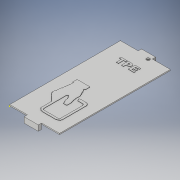
# Autodesk Inventor part: Pièce2
Saved by Autodesk Inventor 2017 (Build 210142000, 142)
## iProperties
Created: 2020-03-28
Part Number: Pièce2
Material: Generic
Document SubType Name: Modeling
Designer: LUC
Density: 1 g/cm^3
Appearance: Default
Author: LUC
Autodesk Inventor part; units mm, degrees
ref_plane "YZ Plane" through (0, 0, 0) normal (1, 0, 0) x (0, 1, 0)
ref_plane "XZ Plane" through (0, 0, 0) normal (0, 1, 0) x (-1, 0, 0)
ref_plane "XY Plane" through (0, 0, 0) normal (0, 0, 1) x (1, 0, 0)
sketch "Esquisse1" plane through (0, 0, 0) normal (0, 1, 0) x (-1, 0, 0)
  point P0 (0, 0)
sketch "Esquisse2" plane through (0, 0, 0) normal (0, 1, 0) x (-1, 0, 0)
  line L0 (0, 0) -> (-45, 0)
  line L1 (-45, 0) -> (-45, -100)
  line L2 (-45, -100) -> (0, -100)
  line L3 (0, -100) -> (0, 0)
  line L4 (-17.07, 0) -> (-29.07, 0)
  line L5 (-17.03, -100) -> (-29.03, -100)
  dimension "d0" = 45
  dimension "d1" = 100
  constraints: 12 end point, 3 horizontal, 2 parallel, 2 point on line, 1 perpendicular
  measures "d0" distance of L2.end L1.end
  measures "d1" distance of L1.end L0.end
extrude "Extrusion1" add sketch "Esquisse2" along normal blind 1
sketch "Esquisse5" plane through (0, 1, 0) normal (0, 1, 0) x (1, 0, 0)
  line L0 (4.5597, 87.1322) -> (40.1621, 87.1322) construction
  line L1 (40.1621, 87.1322) -> (40.1621, 77.2581) construction
  line L2 (40.1621, 77.2581) -> (4.5597, 77.2581) construction
  line L3 (4.5597, 77.2581) -> (4.5597, 87.1322) construction
  line L4 (13.3166, 87.1322) -> (19.0526, 87.1322)
  line L5 (19.0526, 87.1322) -> (19.0526, 85.6234)
  line L6 (19.0526, 85.6234) -> (17.1269, 85.6234)
  line L7 (17.1269, 85.6234) -> (17.1269, 81.0322)
  line L8 (17.1269, 81.0322) -> (15.2423, 81.0322)
  line L9 (15.2423, 81.0322) -> (15.2423, 85.6234)
  line L10 (15.2423, 85.6234) -> (13.3166, 85.6234)
  line L11 (13.3166, 85.6234) -> (13.3166, 87.1322)
  line L12 (19.898, 87.1322) -> (23.0332, 87.1322)
  spline S0 degree 2 poles (23.0332, 87.1322) (24.0547, 87.1322) (25.0763, 86.1576) (25.0763, 85.2594) knots 0 0 0 1 2 2 2
  spline S1 degree 2 poles (25.0763, 85.2594) (25.0763, 84.3317) (23.9667, 83.2926) (22.8277, 83.2926) knots 0 0 0 1 2 2 2
  line L13 (22.8277, 83.2926) -> (21.7944, 83.2926)
  line L14 (21.7944, 83.2926) -> (21.7944, 81.0322)
  line L15 (21.7944, 81.0322) -> (19.898, 81.0322)
  line L16 (19.898, 81.0322) -> (19.898, 87.1322)
  line L17 (21.7944, 84.5313) -> (22.2523, 84.5313)
  spline S2 degree 2 poles (22.2523, 84.5313) (22.7983, 84.5313) (23.2386, 84.913) (23.2386, 85.2065) knots 0 0 0 1 2 2 2
  spline S3 degree 2 poles (23.2386, 85.2065) (23.2386, 85.4942) (22.857, 85.8934) (22.3286, 85.8934) knots 0 0 0 1 2 2 2
  line L18 (22.3286, 85.8934) -> (21.7944, 85.8934)
  line L19 (21.7944, 85.8934) -> (21.7944, 84.5313)
  line L20 (26.0626, 87.1322) -> (31.1117, 87.1322)
  line L21 (31.1117, 87.1322) -> (31.1117, 85.8288)
  line L22 (31.1117, 85.8288) -> (27.9531, 85.8288)
  line L23 (27.9531, 85.8288) -> (27.9531, 84.8601)
  line L24 (27.9531, 84.8601) -> (30.8827, 84.8601)
  line L25 (30.8827, 84.8601) -> (30.8827, 83.6155)
  line L26 (30.8827, 83.6155) -> (27.9531, 83.6155)
  line L27 (27.9531, 83.6155) -> (27.9531, 82.4119)
  line L28 (27.9531, 82.4119) -> (31.2056, 82.4119)
  line L29 (31.2056, 82.4119) -> (31.2056, 81.0322)
  line L30 (31.2056, 81.0322) -> (26.0626, 81.0322)
  line L31 (26.0626, 81.0322) -> (26.0626, 87.1322)
  point P0 (0, 0)
  constraints: 2 other
sketch "Esquisse7" plane through (0, 1, 0) normal (0, 1, 0) x (1, 0, 0)
  line L0 (21.7399, 49.8058) -> (11.605, 49.8058)
  line L1 (11.605, 49.8058) -> (11.605, 49.5446)
  line L2 (11.605, 49.5446) -> (11.309, 49.5446)
  line L3 (11.309, 49.5446) -> (11.309, 49.1789)
  line L4 (11.309, 49.1789) -> (10.9955, 49.1789)
  line L5 (10.9955, 49.1789) -> (10.9955, 45.9399)
  line L6 (10.9955, 45.9399) -> (11.309, 45.9399)
  line L7 (11.309, 45.9399) -> (11.309, 45.6439)
  line L8 (11.309, 45.6439) -> (11.9185, 45.6439)
  line L9 (11.9185, 45.6439) -> (11.9185, 42.4572)
  line L10 (11.9185, 42.4572) -> (11.605, 42.4572)
  line L11 (11.605, 42.4572) -> (11.605, 40.5939)
  line L12 (11.605, 40.5939) -> (11.309, 40.5939)
  line L13 (11.309, 40.5939) -> (11.309, 38.6435)
  line L14 (11.309, 38.6435) -> (10.9955, 38.6435)
  line L15 (10.9955, 38.6435) -> (10.9955, 36.7595)
  line L16 (10.9955, 36.7595) -> (10.9955, 36.3411)
  line L17 (10.9955, 36.3411) -> (10.6437, 36.3411)
  line L18 (10.6437, 36.3411) -> (10.6437, 34.6078)
  line L19 (10.6437, 34.6078) -> (10.315, 34.6078)
  line L20 (10.315, 34.6078) -> (10.315, 32.9043)
  line L21 (10.315, 32.9043) -> (10.315, 31.5295)
  line L22 (10.315, 31.5295) -> (10.046, 31.5295)
  line L23 (10.046, 31.5295) -> (10.046, 30.9617)
  line L24 (10.046, 30.9617) -> (9.6276, 30.9617)
  line L25 (9.6276, 30.9617) -> (9.6276, 28.5111)
  line L26 (9.6276, 28.5111) -> (10.046, 28.5111)
  line L27 (10.046, 28.5111) -> (10.046, 28.003)
  line L28 (10.046, 28.003) -> (10.315, 28.003)
  line L29 (10.315, 28.003) -> (10.315, 27.3754)
  line L30 (10.315, 27.3754) -> (10.6437, 27.3754)
  line L31 (10.6437, 27.3754) -> (10.6437, 26.957)
  line L32 (10.6437, 26.957) -> (10.9955, 26.957)
  line L33 (10.9955, 26.957) -> (10.9955, 26.5984)
  line L34 (10.9955, 26.5984) -> (11.309, 26.5984)
  line L35 (11.309, 26.5984) -> (11.309, 26.1755)
  line L36 (11.309, 26.1755) -> (11.605, 26.1755)
  line L37 (11.605, 26.1755) -> (11.605, 25.8759)
  line L38 (11.605, 25.8759) -> (11.9185, 25.8759)
  line L39 (11.9185, 25.8759) -> (11.9185, 25.5291)
  line L40 (11.9185, 25.5291) -> (12.2466, 25.5291)
  line L41 (12.2466, 25.5291) -> (12.2466, 25.2575)
  line L42 (12.2466, 25.2575) -> (12.5562, 25.2575)
  line L43 (12.5562, 25.2575) -> (12.5562, 24.9339)
  line L44 (12.5562, 24.9339) -> (12.9079, 24.9339)
  line L45 (12.9079, 24.9339) -> (12.9079, 24.6525)
  line L46 (12.9079, 24.6525) -> (13.2175, 24.6525)
  line L47 (13.2175, 24.6525) -> (13.2175, 24.3007)
  line L48 (13.2175, 24.3007) -> (13.5411, 24.3007)
  line L49 (13.5411, 24.3007) -> (13.5411, 24.0193)
  line L50 (13.5411, 24.0193) -> (13.8225, 24.0193)
  line L51 (13.8225, 24.0193) -> (13.8225, 23.6957)
  line L52 (13.8225, 23.6957) -> (14.1883, 23.6957)
  line L53 (14.1883, 23.6957) -> (14.1883, 23.3862)
  line L54 (14.1883, 23.3862) -> (14.4979, 23.3862)
  line L55 (14.4979, 23.3862) -> (14.4979, 23.1329)
  line L56 (14.4979, 23.1329) -> (14.8074, 23.1329)
  line L57 (14.8074, 23.1329) -> (14.8074, 22.7389)
  line L58 (14.8074, 22.7389) -> (15.1029, 22.7389)
  line L59 (15.1029, 22.7389) -> (15.1029, 22.3872)
  line L60 (15.1029, 22.3872) -> (15.4687, 22.3872)
  line L61 (15.4687, 22.3872) -> (15.4687, 22.1058)
  line L62 (15.4687, 22.1058) -> (15.7501, 22.1058)
  line L63 (15.7501, 22.1058) -> (15.7501, 21.7399)
  line L64 (15.7501, 21.7399) -> (16.0878, 21.7399)
  line L65 (16.0878, 21.7399) -> (16.0878, 21.4304)
  line L66 (16.0878, 21.4304) -> (16.327, 21.4304)
  line L67 (16.327, 21.4304) -> (16.327, 21.1349)
  line L68 (16.327, 21.1349) -> (16.6724, 21.1349)
  line L69 (16.6724, 21.1349) -> (16.6724, 11.3222)
  line L70 (16.6724, 11.3222) -> (16.9934, 11.3222)
  line L71 (16.9934, 11.3222) -> (16.9934, 10.929)
  line L72 (16.9934, 10.929) -> (17.3843, 10.929)
  line L73 (17.3843, 10.929) -> (17.3843, 10.5721)
  line L74 (17.3843, 10.5721) -> (17.6902, 10.5721)
  line L75 (17.6902, 10.5721) -> (17.6902, 10.2832)
  line L76 (17.6902, 10.2832) -> (18.0641, 10.2832)
  line L77 (18.0641, 10.2832) -> (18.0641, 9.9943)
  line L78 (18.0641, 9.9943) -> (18.387, 9.9943)
  line L79 (18.387, 9.9943) -> (18.387, 9.6714)
  line L80 (18.387, 9.6714) -> (18.625, 9.6714)
  line L81 (18.625, 9.6714) -> (18.625, 9.3825)
  line L82 (18.625, 9.3825) -> (19.9166, 9.3825)
  line L83 (19.9166, 9.3825) -> (19.9166, 9.0596)
  line L84 (19.9166, 9.0596) -> (32.793, 9.0596)
  line L85 (32.793, 9.0596) -> (32.793, 9.3825)
  line L86 (32.793, 9.3825) -> (33.9518, 9.3825)
  line L87 (33.9518, 9.3825) -> (33.9518, 9.6714)
  line L88 (33.9518, 9.6714) -> (34.4661, 9.6714)
  line L89 (34.4661, 9.6714) -> (34.4661, 9.9943)
  line L90 (34.4661, 9.9943) -> (34.8776, 9.9943)
  line L91 (34.8776, 9.9943) -> (34.8776, 10.2832)
  line L92 (34.8776, 10.2832) -> (35.2634, 10.2832)
  line L93 (35.2634, 10.2832) -> (35.2634, 10.5721)
  line L94 (35.2634, 10.5721) -> (35.5205, 10.5721)
  line L95 (35.5205, 10.5721) -> (35.5205, 10.7506)
  line L96 (35.5205, 10.7506) -> (35.5205, 11.5083)
  line L97 (35.5205, 11.5083) -> (35.8034, 11.5083)
  line L98 (35.8034, 11.5083) -> (35.8034, 33.8684)
  line L99 (35.8034, 33.8684) -> (35.5205, 33.8684)
  line L100 (35.5205, 33.8684) -> (35.5205, 34.6078)
  line L101 (35.5205, 34.6078) -> (35.2634, 34.6078)
  line L102 (35.2634, 34.6078) -> (35.2634, 34.8498)
  line L103 (35.2634, 34.8498) -> (34.8776, 34.8498)
  line L104 (34.8776, 34.8498) -> (34.8776, 35.2086)
  line L105 (34.8776, 35.2086) -> (34.6719, 35.2086)
  line L106 (34.6719, 35.2086) -> (34.6719, 35.4745)
  line L107 (34.6719, 35.4745) -> (33.3724, 35.4745)
  line L108 (33.3724, 35.4745) -> (33.3724, 35.8589)
  line L109 (33.3724, 35.8589) -> (27.4994, 35.8589)
  line L110 (27.4994, 35.8589) -> (27.4994, 35.4745)
  line L111 (27.4994, 35.4745) -> (27.1406, 35.4745)
  line L112 (27.1406, 35.4745) -> (27.1406, 35.0292)
  line L113 (27.1406, 35.0292) -> (27.4994, 35.0292)
  line L114 (27.4994, 35.0292) -> (27.4994, 33.8684)
  line L115 (28.06, 33.8684) -> (28.1721, 33.4596)
  line L116 (28.1721, 33.4596) -> (32.9708, 33.4596)
  line L117 (32.9708, 33.4596) -> (32.9708, 33.2578)
  line L118 (32.9708, 33.2578) -> (33.2174, 33.2578)
  line L119 (33.2174, 33.2578) -> (33.2174, 32.9043)
  line L120 (33.2174, 32.9043) -> (33.6435, 32.9043)
  line L121 (33.6435, 32.9043) -> (33.6435, 32.2169)
  line L122 (33.6435, 32.2169) -> (33.9518, 32.2169)
  line L123 (33.9518, 32.2169) -> (33.9518, 11.8713)
  line L124 (33.9518, 11.8713) -> (33.6435, 11.8713)
  line L125 (33.6435, 11.8713) -> (33.6435, 11.2079)
  line L126 (33.6435, 11.2079) -> (33.2764, 11.2079)
  line L127 (33.2764, 11.2079) -> (33.2764, 10.929)
  line L128 (33.2764, 10.929) -> (19.5666, 10.929)
  line L129 (19.5666, 10.929) -> (19.5666, 11.2079)
  line L130 (19.5666, 11.2079) -> (19.2708, 11.2079)
  line L131 (19.2708, 11.2079) -> (19.2708, 11.5396)
  line L132 (19.2708, 11.5396) -> (18.9755, 11.5396)
  line L133 (18.9755, 11.5396) -> (18.9755, 12.1696)
  line L134 (18.9755, 12.1696) -> (18.625, 12.1696)
  line L135 (18.625, 12.1696) -> (18.625, 32.5606)
  line L136 (18.625, 32.5606) -> (18.9755, 32.5606)
  line L137 (18.9755, 32.5606) -> (18.9755, 32.9043)
  line L138 (18.9755, 32.9043) -> (18.9755, 33.2578)
  line L139 (18.9755, 33.2578) -> (19.5666, 33.2399)
  line L140 (19.5666, 33.2399) -> (19.5666, 33.5677)
  line L141 (19.5666, 33.5677) -> (19.8877, 33.5677)
  line L142 (19.8877, 33.5677) -> (19.8877, 32.9043)
  line L143 (19.8877, 32.9043) -> (20.1961, 32.9043)
  line L144 (20.1961, 32.9043) -> (20.1961, 32.5606)
  line L145 (20.1961, 32.5606) -> (20.5094, 32.5606)
  line L146 (20.5094, 32.5606) -> (20.5094, 31.9807)
  line L147 (20.5094, 31.9807) -> (21.149, 31.9807)
  line L148 (21.149, 31.9807) -> (21.149, 31.3486)
  line L149 (21.149, 31.3486) -> (21.5008, 31.3486)
  line L150 (21.5008, 31.3486) -> (21.5008, 30.6609)
  line L151 (21.5008, 30.6609) -> (21.784, 30.6609)
  line L152 (21.784, 30.6609) -> (21.784, 28.4465)
  line L153 (21.784, 28.4465) -> (22.1511, 28.4465)
  line L154 (22.1511, 28.4465) -> (22.1511, 27.5143)
  line L155 (22.1511, 27.5143) -> (22.4573, 27.5143)
  line L156 (22.4573, 27.5143) -> (22.4573, 26.871)
  line L157 (22.4573, 26.871) -> (22.7348, 26.871)
  line L158 (22.7348, 26.871) -> (22.7348, 26.5304)
  line L159 (22.7348, 26.5304) -> (23.088, 26.5304)
  line L160 (23.088, 26.5304) -> (23.088, 25.8759)
  line L161 (23.088, 25.8759) -> (23.416, 25.8759)
  line L162 (23.416, 25.8759) -> (23.416, 25.2575)
  line L163 (23.416, 25.2575) -> (23.7313, 25.2575)
  line L164 (23.7313, 25.2575) -> (23.7313, 24.9339)
  line L165 (23.7313, 24.9339) -> (26.2794, 24.9339)
  line L166 (26.2794, 24.9339) -> (26.2794, 25.5667)
  line L167 (26.2794, 25.5667) -> (26.5845, 25.5667)
  line L168 (26.5845, 25.5667) -> (26.5845, 29.0911)
  line L169 (26.5845, 29.0911) -> (26.2794, 29.0911)
  line L170 (26.2794, 29.0911) -> (26.2794, 30.3514)
  line L171 (26.2794, 30.3514) -> (25.9641, 30.3514)
  line L172 (25.9641, 30.3514) -> (25.9641, 31.6647)
  line L173 (25.9641, 31.6647) -> (25.5856, 31.6647)
  line L174 (25.5856, 31.6647) -> (25.5856, 33.8684)
  line L175 (25.5856, 33.8684) -> (25.2829, 33.8684)
  line L176 (25.2829, 33.8684) -> (25.2829, 38.6435)
  line L177 (25.2829, 38.6435) -> (25.0054, 38.6435)
  line L178 (25.0054, 38.6435) -> (25.0054, 39.2708)
  line L179 (25.0054, 39.2708) -> (24.6774, 39.2708)
  line L180 (24.6774, 39.2708) -> (24.6774, 40.3012)
  line L181 (24.6774, 40.3012) -> (24.4084, 40.3012)
  line L182 (24.4084, 40.3012) -> (24.4084, 40.9021)
  line L183 (24.4084, 40.9021) -> (24.0221, 40.9021)
  line L184 (24.0221, 40.9021) -> (24.0221, 41.2311)
  line L185 (24.0221, 41.2311) -> (23.7313, 41.2311)
  line L186 (23.7313, 41.2311) -> (23.7313, 41.8463)
  line L187 (23.7313, 41.8463) -> (23.416, 41.8463)
  line L188 (23.416, 41.8463) -> (23.416, 42.8192)
  line L189 (23.416, 42.8192) -> (23.088, 42.8192)
  line L190 (23.088, 42.8192) -> (23.088, 43.1196)
  line L191 (23.088, 43.1196) -> (22.7348, 43.1196)
  line L192 (22.7348, 43.1196) -> (22.7348, 43.7491)
  line L193 (22.7348, 43.7491) -> (22.4573, 43.7491)
  line L194 (22.4573, 43.7491) -> (22.4573, 44.0505)
  line L195 (22.4573, 44.0505) -> (22.1511, 44.0505)
  line L196 (22.1511, 44.0505) -> (22.1511, 44.4072)
  line L197 (22.1511, 44.4072) -> (21.8618, 44.4072)
  line L198 (21.8618, 44.4072) -> (21.8618, 45.3229)
  line L199 (21.8618, 45.3229) -> (22.1511, 45.3229)
  line L200 (22.1511, 45.3229) -> (22.1511, 45.6439)
  line L201 (22.1511, 45.6439) -> (22.7348, 45.6439)
  line L202 (22.7348, 45.6439) -> (22.7348, 49.5446)
  line L203 (22.7348, 49.5446) -> (22.1511, 49.5446)
  line L204 (22.1511, 49.5446) -> (22.1511, 49.8058)
  line L205 (22.1511, 49.8058) -> (21.7399, 49.8058)
  line L206 (28.06, 33.8684) -> (27.4994, 33.8684)
  point P0 (0, 0)
  constraints: 414 end point, 168 perpendicular, 58 point on line, 5 vertical, 3 horizontal
extrude "Extrusion3" add sketch "Esquisse5" along normal blind 0.3
extrude "Extrusion4" add sketch "Esquisse7" along normal blind 0.3
sketch "Esquisse14" plane through (0, 1, 0) normal (0, 1, 0) x (1, 0, 0)
  line L0 (16, 100) -> (28.8, 100)
  line L1 (28.8, 100) -> (28.8, 103)
  line L2 (28.8, 103) -> (16, 103)
  line L3 (16, 103) -> (16, 100)
  line L4 (0, 100) -> (0, 0) projected
  line L5 (16, 0) -> (28.8, 0)
  line L6 (28.8, 0) -> (28.8, -3)
  line L7 (28.8, -3) -> (16, -3)
  line L8 (16, -3) -> (16, 0)
  dimension "d47" = 12.8
  dimension "d48" = 3
  dimension "d49" = 16
  dimension "d50" = 12.8
  dimension "d51" = 3
  constraints: 16 end point, 4 parallel, 2 horizontal, 2 perpendicular
  measures "d47" distance of L2.end L1.end
  measures "d48" distance of L1.end L0.end
  measures "d49" distance from line of L4 L0.start
  measures "d50" distance of L6.end L7.end
  measures "d51" distance of L5.end L6.end
extrude "Extrusion8" add sketch "Esquisse14" against normal blind 5
sketch "Esquisse15" plane through (0, 1, 0) normal (0, 1, 0) x (1, 0, 0)
  line L0 (45, 100) -> (28.8, 100) projected
  line L1 (45, 100) -> (27, 100)
  line L2 (27, 100) -> (27, 98)
  line L3 (27, 98) -> (45, 98)
  line L4 (45, 98) -> (45, 100)
  point P0 (0, 0)
  dimension "d54" = 18
  dimension "d55" = 2
  constraints: 8 end point, 2 parallel, 1 horizontal, 1 perpendicular
  measures "d54" distance of L3.end L2.end
  measures "d55" distance of L2.end L1.end
hole "Perçage2" at (27, 1, -98) direction (0, -1, 0) diameter 3 end through all
